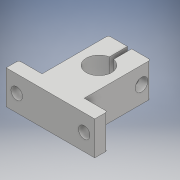
# Autodesk Inventor part: Sk12
Saved by Autodesk Inventor 2018 (Build 220112000, 112)
## iProperties
Created: 2018-09-20
Part Number: Sk12
Material: Genérico
Document SubType Name: Modeling
Designer: Georgines
Density: 1 g/cm^3
Appearance: Padrão
Author: Georgines
Autodesk Inventor part; units mm, degrees
ref_plane "YZ Plane" through (0, 0, 0) normal (1, 0, 0) x (0, 1, 0)
ref_plane "XZ Plane" through (0, 0, 0) normal (0, 1, 0) x (-1, 0, 0)
ref_plane "XY Plane" through (0, 0, 0) normal (0, 0, 1) x (1, 0, 0)
sketch "Esboço1" plane through (0, 0, 0) normal (0, 0, 1) x (1, 0, 0)
  line L0 (17.7277, 1.9549) -> (-24.2723, 1.9549)
  line L1 (-24.2723, 1.9549) -> (-24.2723, 7.9549)
  line L2 (17.7277, 7.9549) -> (17.7277, 1.9549)
  line L3 (6.7277, 39.4549) -> (6.7277, 7.9549)
  line L4 (-13.2723, 7.9549) -> (-13.2723, 39.4549)
  arc A0 (-4.2723, 30.871) -> (-2.2723, 30.871) centre (-3.2723, 24.9549) ccw
  line L5 (-24.2723, 7.9549) -> (-13.2723, 7.9549)
  line L6 (6.7277, 7.9549) -> (17.7277, 7.9549)
  line L7 (-2.2723, 39.4549) -> (-2.2723, 30.871)
  line L8 (-4.2723, 30.871) -> (-4.2723, 39.4549)
  line L9 (-13.2723, 39.4549) -> (-4.2723, 39.4549)
  line L10 (-2.2723, 39.4549) -> (6.7277, 39.4549)
  dimension "largura" = 42
  dimension "largura_topo" = 20
  dimension "altura_base" = 6
  dimension "diametro" = 12
  dimension "altura_furo" = 23
  dimension "d6" = 11
  dimension "d7" = 10
  dimension "d8" = 6
  dimension "d10" = 9
  dimension "d11" = 9
  dimension "altura" = 37.5
  dimension "d33" = 37.5
  constraints: 22 end point, 5 parallel, 4 perpendicular, 3 horizontal, 2 point on circle, 1 centre point
  measures "largura" distance of L0.start L0.end
  measures "largura_topo" distance of L4.end L3.start
  measures "altura_base" distance of L0.end L1.end
  measures "diametro" diameter of A0
  measures "altura_furo" distance from line of A0.centre L0
  measures "d6" distance of L1.end L4.start
  measures "d7" distance from line of L4 A0.centre
  measures "d8" distance of L2.start L0.start
  measures "d10" distance of L7.start L3.start
  measures "d11" distance of L4.end L8.end
  measures "altura" distance between parallel lines of L0 L10
  measures "d33" distance between parallel lines of L0 L9
extrude "Extrusão1" add sketch "Esboço1" along normal blind 16
sketch "Esboço2" plane through (6.7277, 7.9549, 0) normal (1, 0, 0) x (0, 0, -1)
  line L0 (0, 22.9161) -> (-16, 22.9161) projected
  line L1 (-8, 22.9161) -> (-8, 31.5) construction
  circle A0 centre (-8, 27.208) radius 1.1711 construction
  line L2 (0, 31.5) -> (-16, 31.5) projected
  point P0 (0, -7.9549)
  constraints: 3 midpoint, 2 end point, 1 centre point, 1 vertical
hole "Furo1" at (6.7277, 35.163, 8) direction (-1, 0, 0) diameter 3.242 end through all counterbore diameter 6 counterbore depth 4 thread size "M4x0.7" class "6H" standard "ANSI Metric M Profile"
sketch "Esboço3" plane through (-24.2723, 1.9549, 0) normal (0, -1, 0) x (1, 0, 0)
  line L0 (5, 8) -> (37, 8) construction
  circle A0 centre (5, 8) radius 1 construction
  circle A1 centre (37, 8) radius 1 construction
  line L1 (42, 0) -> (0, 0) construction
  line L2 (21, 0) -> (21, 16) construction
  line L3 (0, 16) -> (42, 16) construction
  point P0 (21, 8)
  dimension "distancia_parafusos" = 32
  dimension "d22" = 2
  dimension "d23" = 2
  constraints: 4 end point, 4 midpoint, 2 centre point, 2 coincident, 1 horizontal
  measures "distancia_parafusos" distance of L0.start L0.end
  measures "d22" diameter of A0
  measures "d23" diameter of A1
hole "Furo2" at (-19.2723, 1.9549, 8) at (12.7277, 1.9549, 8) direction (0, 1, 0) diameter 5.5 end through all
fillet "Arredondamento1" radius 1 4 edges at (6.7277, 39.4549, 8) (-13.2723, 39.4549, 8) (-24.2723, 7.9549, 8) (17.7277, 7.9549, 8)
equation "\"d6\" = -0.5 * largura_topo + 0.5 * largura"
equation "\"d7\" = 0.5 * largura_topo"
equation "\"d8\" = altura_base"
equation "\"d11\" = d10"
equation "\"d33\" = altura"
